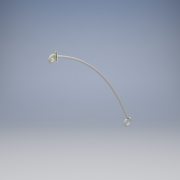
# Autodesk Inventor part: 123
Saved by Autodesk Inventor 2018 (Build 220112000, 112)
## iProperties
Created: 2019-05-31
Part Number: 123
Material: Generic
Document SubType Name: Modeling
Designer: ch1180207
Density: 1 g/cm^3
Appearance: Default
Author: ch1180207
Autodesk Inventor part; units mm, degrees
ref_plane "YZ Plane" through (0, 0, 0) normal (1, 0, 0) x (0, 1, 0)
sketch "Sketch1" plane through (0, 0, 0) normal (0, 1, 0) x (-1, 0, 0)
  circle A0 centre (0, 30) radius 10
  line L0 (14, 0) -> (-14, 0) projected
  point P0 (0, 0)
  dimension "d0" = 20
  constraints: 1 centre point
  measures "d0" diameter of A0
revolve "Revolution1" add sketch "Sketch1" angle 360 about axis through (-10, 0, 0) along (1, 0, 0)
sketch "Sketch2" plane through (0, 0, 0) normal (1, 0, 0) x (0, 1, 0)
  point P0 (0, 0)
ref_plane "Work Plane1" through (0, 400, 0) normal (0, 1, 0) x (-1, 0, 0)
ref_plane "Work Plane2" through (0, 40, 0) normal (0, 1, 0) x (-1, 0, 0)
sketch "Sketch3" plane through (0, 40, 0) normal (0, 1, 0) x (-1, 0, 0)
  circle A0 centre (0, 0) radius 10
  dimension "d4" = 20
  constraints: 1 centre point, 1 coincident
  measures "d4" diameter of A0
sketch "Sketch4" plane through (0, 0, 0) normal (1, 0, 0) x (0, 1, 0)
  line L0 (40.139, 0) -> (545.4376, -248.5404) construction
  line L1 (545.4376, -248.5404) -> (800, -950) construction
  spline S0 degree 2 poles (40.139, 0) (545.4376, -248.5404) (800, -950) knots 1 1 1 2 2 2
  point P0 (0, 0)
  point P1 (950, 800)
  constraints: 3 other
sweep "Sweep1" add profiles "Sketch3" path "Sketch4"
ref_plane "Work Plane3" through (0, 800, 0) normal (0, 1, 0) x (-1, 0, 0)
sketch "Sketch5" plane through (0, 800, 0) normal (0, 1, 0) x (-1, 0, 0)
  line L0 (0, -979.563) -> (19.5024, -979.563)
  circle A0 centre (0, -949.5625) radius 10
  point P0 (0, 0)
  dimension "d8" = 20
  constraints: 2 end point, 1 centre point, 1 coincident, 1 horizontal
  measures "d8" diameter of A0
revolve "Revolution2" add sketch "Sketch5" angle 360 about axis through (0, 800, -979.563) along (-1, 0, 0)
body "Solid1"
